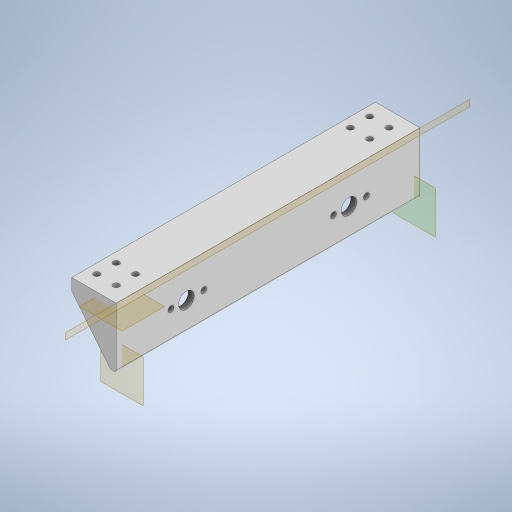
# Autodesk Inventor part: крепёж_мотора_f
Saved by Autodesk Inventor 2023 (Build 270158000, 158)
## iProperties
Created: 2025-12-12
Part Number: крепёж_мотора_f
Material: Типовые
Document SubType Name: Modeling
Designer: garin
Density: 1 g/cm^3
Appearance: По умолчанию
Author: garin
Autodesk Inventor part; units mm, degrees
ref_plane "YZ Plane" through (0, 0, 0) normal (1, 0, 0) x (0, 1, 0)
ref_plane "XZ Plane" through (0, 0, 0) normal (0, 1, 0) x (-1, 0, 0)
ref_plane "XY Plane" through (0, 0, 0) normal (0, 0, 1) x (1, 0, 0)
ref_plane "РабПлоскость1" through (57.3886, 15.9976, 24.7396) normal (1, 0, 0) x (0, 1, 0)
sketch "Эскиз1" plane through (57.3886, 15.9976, 24.7396) normal (1, 0, 0) x (0, 1, 0)
  circle A0 centre (-16.5, 48) radius 1.5
  circle A1 centre (-16.5, 31) radius 1.5
  circle A2 centre (-16.5, 40) radius 4
  circle A3 centre (-16.5, 40) radius 12.75
  circle A4 centre (-16.5, 132) radius 1.5
  circle A5 centre (-16.5, 115) radius 1.5
  circle A6 centre (-16.5, 124) radius 4
  circle A7 centre (-16.5, 124) radius 12.75
  line L0 (-3.75, 40) -> (-2.75, 40)
  line L1 (-30.75, 6.25) -> (-30.75, 157.25)
  line L2 (-30.75, 157.25) -> (-2.75, 157.25)
  line L3 (-30.75, 6.25) -> (0.25, 6.25)
  line L4 (0.25, 6.25) -> (0.25, 157.25)
  line L5 (0.25, 157.25) -> (-30.75, 157.25)
  line L6 (-30.75, 157.25) -> (-30.75, 6.25)
  point P0 (-15.9976, -24.7396)
  point P1 (-15.5, 28.25)
  point P2 (-2.75, 157.25)
  dimension "d15" = 25.5
  dimension "d43" = 25.5
  dimension "d44" = 1
  dimension "d45" = 28
  dimension "d46" = 151
  dimension "d79" = 31
  constraints: 14 end point, 7 centre point, 2 coincident, 2 horizontal, 2 parallel, 1 horizontal alignment, 1 perpendicular, 2 other
  measures "d43" diameter of A7
  measures "d44" distance of L0.start L0.end
  measures "d45" distance of L1.end L2.end
  measures "d46" distance of L1.start L1.end
  measures "d79" distance of L5.end L4.end
ref_plane "РабПлоскость2" through (57.3886, 13.2476, 181.9896) normal (0, 1, 0) x (1, 0, 0)
sketch "Эскиз5" plane through (57.3886, 13.2476, 181.9896) normal (0, 1, 0) x (1, 0, 0)
  line L0 (-3, 0) -> (-23, 0)
  line L1 (-23, 0) -> (-23, 20)
  line L2 (-3, 20) -> (-3, 0)
  line L3 (-3, 151) -> (-3, 0) projected
  line L4 (-23, 0) -> (-3, 0)
  line L5 (-3, 0) -> (-3, 5)
  line L6 (-23, 5) -> (-23, 0)
  line L7 (-23, 0) -> (-18, 0)
  line L8 (-23, 20) -> (-23, 0)
  line L9 (-3, 20) -> (-3, 15)
  line L10 (-23, 15) -> (-23, 20)
  line L11 (-8, 0) -> (-3, 0)
  line L12 (-3, 0) -> (-3, 20)
  circle A0 centre (-18, 5) radius 1.5
  circle A1 centre (-18, 15) radius 1.5
  circle A2 centre (-8, 15) radius 1.5
  circle A3 centre (-8, 5) radius 1.5
  line L13 (-3, 151) -> (-23, 151)
  line L14 (-23, 151) -> (-23, 131)
  line L15 (-3, 131) -> (-3, 151)
  line L16 (-3, 151) -> (-23, 151)
  line L17 (-23, 151) -> (-23, 146)
  line L18 (-3, 146) -> (-3, 151)
  line L19 (-23, 151) -> (-18, 151)
  line L20 (-23, 131) -> (-23, 151)
  line L21 (-3, 131) -> (-3, 136)
  line L22 (-23, 136) -> (-23, 131)
  line L23 (-8, 151) -> (-3, 151)
  line L24 (-3, 151) -> (-3, 131)
  circle A4 centre (-18, 136) radius 1.5
  circle A5 centre (-18, 146) radius 1.5
  circle A6 centre (-8, 146) radius 1.5
  circle A7 centre (-8, 136) radius 1.5
  line L25 (-23, 20) -> (-23, 131)
  line L26 (-3, 20) -> (-3, 131)
  point P0 (-57.3886, 181.9896)
  point P1 (-23, 131)
  constraints: 52 end point, 8 centre point, 6 horizontal, 6 parallel, 6 point on line, 4 perpendicular, 1 collinear, 1 vertical
ref_plane "РабПлоскость3" through (57.3886, -14.7524, 181.9896) normal (0, 0, 1) x (1, 0, 0)
sketch "Эскиз6" plane through (57.3886, -14.7524, 181.9896) normal (0, 0, 1) x (1, 0, 0)
  line L0 (-3, 28) -> (-23, 28) projected
  line L1 (-3, 25) -> (-23, 25) projected
  line L2 (-23, 28) -> (-23, 25)
  line L3 (0, 0) -> (-3, 0) projected
  line L4 (-23, 25) -> (-3, 0)
  line L5 (-3, 0) -> (0, 0)
  line L6 (0, 28) -> (0, 0) projected
  line L7 (0, 0) -> (0, 28)
  line L8 (0, 28) -> (-23, 28)
  point P0 (-57.3886, 14.7524)
  constraints: 10 end point, 2 perpendicular, 1 collinear, 1 vertical
ref_plane "РабПлоскость4" through (57.3886, -14.7524, 30.9896) normal (0, 0, -1) x (-1, 0, 0)
sketch "Эскиз7" plane through (57.3886, -14.7524, 30.9896) normal (0, 0, -1) x (-1, 0, 0)
  line L0 (0, 28) -> (0, 0) projected
  line L1 (3, 28) -> (23, 28) projected
  line L2 (0, 28) -> (23, 28)
  line L3 (3, 25) -> (23, 25) projected
  line L4 (23, 28) -> (23, 25)
  line L5 (0, 0) -> (3, 0) projected
  line L6 (23, 25) -> (3, 0)
  line L7 (3, 0) -> (0, 0)
  line L8 (0, 0) -> (0, 28)
  point P0 (57.3886, 14.7524)
  constraints: 10 end point, 2 perpendicular, 1 horizontal, 1 parallel
extrude "Выдавливание8" add sketch "Эскиз7" along normal blind 3
extrude "Выдавливание9" add sketch "Эскиз6" along normal blind 3
extrude "Выдавливание10" add sketch "Эскиз1" against normal blind 3 contours A3 | A7 | L1 L2 L5 L4 L3
extrude "Выдавливание11" add sketch "Эскиз5" along normal blind 3
sketch "Эскиз8" plane through (57.3886, 16.2476, 181.9896) normal (0, 1, 0) x (1, 0, 0)
  line L0 (0, 151) -> (0, 154) projected
  line L1 (-23, 154) -> (0, 154) projected
  line L2 (0, 151) -> (-23, 151)
  line L3 (-23, 151) -> (-23, 154)
  line L4 (-23, 154) -> (0, 154)
  line L5 (0, 154) -> (0, 151)
  line L6 (0, 0) -> (0, -3) projected
  line L7 (0, -3) -> (-23, -3) projected
  line L8 (0, 0) -> (-23, 0)
  line L9 (-23, 0) -> (-23, -3)
  line L10 (-23, -3) -> (0, -3)
  line L11 (0, -3) -> (0, 0)
  point P0 (-57.3886, 181.9896)
  constraints: 16 end point, 4 parallel, 2 horizontal, 2 perpendicular
extrude "Выдавливание12" add sketch "Эскиз8" against normal blind 3
fillet "Сопряжение7" radius 1 1 edges at (57.3886, -14.7524, 106.4896)
fillet "Сопряжение8" radius 1 1 edges at (54.3886, -14.7524, 106.4896)
fillet "Сопряжение9" radius 2 1 edges at (54.3886, -14.7524, 183.4896)
fillet "Сопряжение10" radius 2 1 edges at (54.3886, -14.7524, 29.4896)
